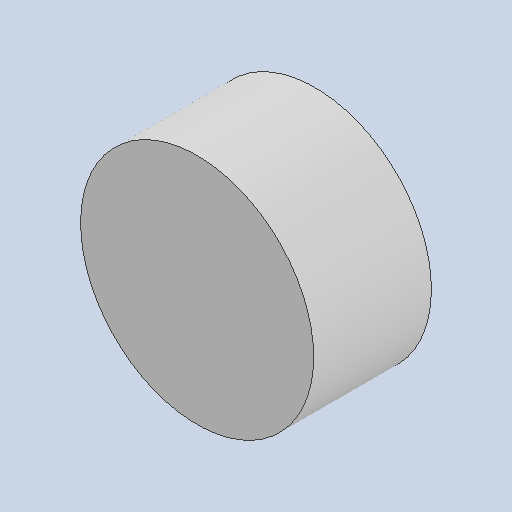
# Autodesk Inventor part: TTencoderspacer
Saved by Autodesk Inventor 2022 (Build 260153070, 153G)
## iProperties
Created: 2021-11-27
Part Number: TTencoderspacer
Material: Generic
Document SubType Name: Modeling
Designer: a laptop
Density: 1 g/cm^3
Appearance: Default
Author: a laptop
Autodesk Inventor part; units mm, degrees
ref_plane "YZ Plane" through (0, 0, 0) normal (1, 0, 0) x (0, 1, 0)
ref_plane "XZ Plane" through (0, 0, 0) normal (0, 1, 0) x (-1, 0, 0)
sketch "Sketch1" plane through (0, 0, 0) normal (0, 0, 1) x (1, 0, 0)
  line L0 (2.6366, 1.85) -> (-1.2966, 1.85) construction
  arc A0 (-1.2966, 1.85) -> (-1.2966, -1.85) centre (0.67, 0) ccw construction
  arc A1 (2.6366, -1.85) -> (2.6366, 1.85) centre (0.67, 0) ccw construction
  line L1 (-1.2966, -1.85) -> (2.6366, -1.85) construction
  circle A2 centre (0.67, 0) radius 4.7
  arc A3 (-1.3604, 2) -> (-1.3604, 2) centre (0.67, 0) ccw
  line L2 (-1.3604, 2) -> (2.7004, 2)
  line L3 (-1.3604, 2) -> (2.7004, 2)
  arc A4 (2.7004, 2) -> (2.7004, 2) centre (0.67, 0) ccw
  point P0 (0, 0)
  dimension "d0" = 2
  dimension "d6" = 0.15
  dimension "d7" = 0.15
  constraints: 4 concentric, 4 end point, 4 point on circle, 3 centre point, 2 collinear, 1 coincident, 1 horizontal
  measures "d0" radial gap between concentric circles of A2 A0
  measures "d6" distance between parallel lines of L0 L2
  measures "d7" radial gap between concentric circles of A3 A0
ref_plane "Work Plane1" through (-12.875, -12.875, 4.75) normal (0, 0, -1) x (0, 1, 0)
extrude "Extrusion1" add sketch "Sketch1" along normal up to surface (4.75 mm away) contours A2 | A3 L2 | L2 A3
body "Solid1"
